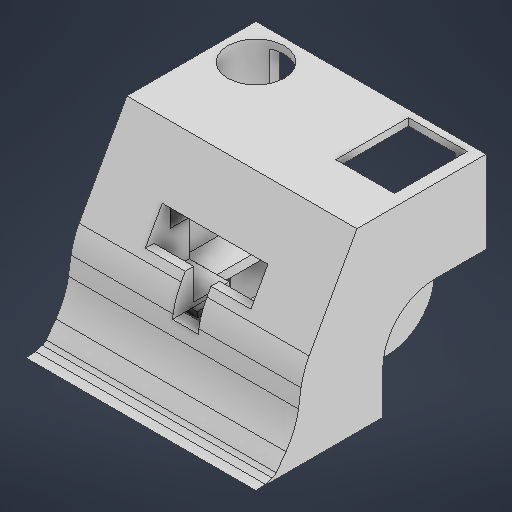
# Autodesk Inventor part: najlepszetrzecieniepierwszekolokwium
Saved by Autodesk Inventor 2026 (Build 300175000, 175)
## iProperties
Created: 2025-12-31
Part Number: najlepszetrzecieniepierwszekolokwium
Material: Ogólny
Document SubType Name: Modeling
Designer: macie
Density: 1 g/cm^3
Appearance: Domyślna
Author: macie
Autodesk Inventor part; units mm, degrees
ref_plane "YZ Plane" through (0, 0, 0) normal (1, 0, 0) x (0, 1, 0)
ref_plane "XZ Plane" through (0, 0, 0) normal (0, 1, 0) x (-1, 0, 0)
ref_plane "XY Plane" through (0, 0, 0) normal (0, 0, 1) x (1, 0, 0)
sketch "Szkic1" plane through (0, 0, 0) normal (0, 1, 0) x (-1, 0, 0)
  line L0 (49, 49) -> (-49, 49)
  line L1 (-49, 49) -> (-49, -49)
  line L2 (-49, -49) -> (49, -49)
  line L3 (49, -49) -> (49, 49)
  line L4 (49, 49) -> (-49, -49) construction
  line L5 (-49, 49) -> (49, -49) construction
  point P0 (0, 0)
  dimension "d0" = 98
  dimension "d1" = 98
  constraints: 12 end point, 2 midpoint, 2 parallel, 1 horizontal, 1 perpendicular
  measures "d0" distance between parallel lines of L1 L3
  measures "d1" distance between parallel lines of L2 L0
extrude "Wyciągnięcie proste1" add sketch "Szkic1" along normal blind 98
sketch "Szkic2" plane through (49, 0, 49) normal (1, 0, 0) x (0, 0, -1)
  line L0 (0, 0) -> (98, 0) projected
  line L1 (98, 0) -> (76, 0)
  line L2 (76, 0) -> (76, 18)
  circle A0 centre (76, 18) radius 22
  line L3 (98, 0) -> (98, 98) projected
  line L4 (98, 18) -> (98, 0)
  line L5 (98, 0) -> (88.6491, 0)
  line L6 (76, 40) -> (98, 40)
  line L7 (98, 18) -> (98, 40)
  line L8 (54, 18) -> (54, 0)
  line L9 (63.3509, 0) -> (54, 0)
  point P0 (49, 0)
  dimension "d4" = 22
  dimension "d5" = 18
  dimension "d6" = 44
  constraints: 16 end point, 6 point on line, 5 point on circle, 2 collinear, 2 perpendicular, 2 tangent, 2 vertical, 1 centre point, 1 coincident
  measures "d4" distance of L0.end L1.end
  measures "d5" distance of L1.end L2.end
  measures "d6" diameter of A0
extrude "Wyciągnięcie proste2" cut sketch "Szkic2" against normal blind 98 contours L8 A0 L0 | A0 L0 | A0 L3 L0 | L6 L3 A0 picked at (77.6318, 26.4828)
sketch "Szkic3" plane through (0, 0, 0) normal (0, -1, 0) x (1, 0, 0)
  line L0 (49, -49) -> (-49, -49) projected
  line L1 (49, -49) -> (27, -49)
  line L2 (-49, -49) -> (-27, -49)
  line L3 (-49, -5) -> (49, -5) projected
  line L4 (-27, -49) -> (27, -49)
  line L5 (27, -49) -> (27, -5)
  line L6 (27, -5) -> (-27, -5)
  line L7 (-27, -5) -> (-27, -49)
  point P0 (0, 0)
  dimension "d10" = 22
  dimension "d11" = 22
  dimension "d12" = 54
  constraints: 12 end point, 3 point on line, 2 parallel, 1 horizontal, 1 perpendicular
  measures "d10" distance of L1.end L0.start
  measures "d11" distance of L2.end L0.end
  measures "d12" distance between parallel lines of L7 L5
extrude "Wyciągnięcie proste3" add sketch "Szkic3" against normal blind 40
sketch "Szkic4" plane through (27, 0, -5) normal (1, 0, 0) x (0, 0, -1)
  line L0 (44, 0) -> (44, 40) projected
  line L1 (44, 18) -> (44, 0)
  line L2 (44, 18) -> (22, 18)
  line L3 (22, 12) -> (22, 24)
  line L4 (15, 24) -> (29, 24)
  line L5 (15, 24) -> (15, 12)
  line L6 (15, 12) -> (29, 12)
  line L7 (29, 12) -> (29, 24)
  point P0 (-5, 0)
  dimension "d15" = 18
  dimension "d16" = 22
  dimension "d17" = 12
  dimension "d18" = 14
  dimension "d19" = 12
  constraints: 14 end point, 3 vertical, 2 horizontal, 2 midpoint, 2 perpendicular, 1 point on line
  measures "d15" distance of L0.start L1.start
  measures "d16" distance of L1.start L2.end
  measures "d17" distance of L3.start L3.end
  measures "d18" distance of L4.end L4.start
  measures "d19" distance between parallel lines of L4 L6
extrude "Wyciągnięcie proste4" cut sketch "Szkic4" against normal through all
sketch "Szkic5" plane through (49, 98, -49) normal (0, 0, -1) x (-1, 0, 0)
  line L0 (98, 0) -> (0, 0) projected
  line L1 (98, -98) -> (98, 0) projected
  line L2 (0, 0) -> (98, 0)
  line L3 (98, 0) -> (98, -30)
  line L4 (98, -30) -> (0, -30)
  line L5 (0, -30) -> (0, 0)
  line L6 (0, -58) -> (22, -58) projected
  line L7 (10, -58) -> (88, -58)
  line L8 (88, -58) -> (88, -38)
  line L9 (88, -38) -> (10, -38)
  line L10 (10, -38) -> (10, -58)
  line L11 (0, -58) -> (0, 0) projected
  line L12 (22, -86) -> (76, -86) projected
  line L13 (38, -86) -> (60, -86)
  line L14 (60, -86) -> (60, -58)
  line L15 (60, -58) -> (38, -58)
  line L16 (38, -58) -> (38, -86)
  line L17 (22, -98) -> (22, -58) projected
  line L18 (76, -98) -> (76, -58) projected
  line L19 (22, -70) -> (38, -70)
  line L20 (60, -70) -> (76, -70)
  line L21 (76, -70) -> (76, -58)
  line L22 (22, -70) -> (22, -58)
  line L23 (22, -74) -> (76, -74) projected
  line L24 (22, -90) -> (22, -96)
  line L25 (76, -96) -> (22, -96)
  line L26 (76, -96) -> (76, -86)
  line L27 (76, -98) -> (22, -98) projected
  line L28 (22, -96) -> (22, -90)
  line L29 (22, -90) -> (76, -90)
  line L30 (76, -96) -> (76, -90)
  line L31 (38, -86) -> (38, -90)
  line L32 (60, -86) -> (60, -90)
  line L33 (24, -58) -> (24, -70)
  line L34 (74, -58) -> (74, -70)
  line L35 (10, -56) -> (24, -56)
  line L36 (24, -56) -> (24, -58)
  line L37 (74, -58) -> (74, -56)
  line L38 (74, -56) -> (88, -56)
  point P0 (49, -98)
  dimension "d22" = 30
  dimension "d23" = 20
  dimension "d25" = 10
  dimension "d26" = 10
  dimension "d27" = 16
  dimension "d28" = 16
  dimension "d29" = 4
  dimension "d30" = 2
  dimension "d31" = 4
  dimension "d32" = 2
  dimension "d33" = 2
  dimension "d34" = 2
  dimension "d35" = 2
  constraints: 60 end point, 22 point on line, 13 perpendicular, 6 parallel, 5 collinear, 2 horizontal, 1 vertical
  measures "d22" distance between parallel lines of L4 L0
  measures "d23" distance between parallel lines of L7 L9
  measures "d25" distance between parallel lines of L11 L10
  measures "d26" distance between parallel lines of L1 L8
  measures "d27" distance between parallel lines of L17 L16
  measures "d28" distance between parallel lines of L18 L14
  measures "d29" distance between parallel lines of L23 L19
  measures "d30" distance between parallel lines of L27 L25
  measures "d31" distance between parallel lines of L29 L12
  measures "d32" distance between parallel lines of L17 L33
  measures "d33" distance between parallel lines of L34 L18
  measures "d34" distance between parallel lines of L7 L35
  measures "d35" distance between parallel lines of L7 L38
extrude "Wyciągnięcie proste5" cut sketch "Szkic5" against normal blind 55 contours L10 L9 L8 L38 L37 L7 L36 L35 | L7 L16 L19 L33 | L7 L14 L23 L16 | L7 L34 L20 L14 | L23 L14 L12 L16
sketch "Szkic6" plane through (0, 0, 0) normal (0, -1, 0) x (1, 0, 0)
  line L0 (38.5, -16) -> (-38.5, -16)
  line L1 (-38.5, -16) -> (-38.5, 25)
  line L2 (-38.5, 25) -> (38.5, 25)
  line L3 (38.5, 25) -> (38.5, -16)
  line L4 (-49, -5) -> (-49, 49) projected
  line L5 (49, 49) -> (49, -5) projected
  line L6 (27, -5) -> (49, -5) projected
  line L7 (27, -20) -> (11, -20) projected
  point P0 (0, 0)
  dimension "d38" = 41
  dimension "d40" = 10.5
  dimension "d41" = 10.5
  dimension "d45" = 4
  constraints: 8 end point, 2 parallel, 1 horizontal, 1 perpendicular
  measures "d38" distance between parallel lines of L2 L0
  measures "d40" distance between parallel lines of L4 L1
  measures "d41" distance between parallel lines of L3 L5
  measures "d45" distance between parallel lines of L0 L7
extrude "Wyciągnięcie proste6" cut sketch "Szkic6" against normal blind 24
sketch "Szkic7" plane through (0, 0, 0) normal (0, -1, 0) x (1, 0, 0)
  line L0 (-38.5, 25) -> (38.5, 25) projected
  line L1 (38.5, 25) -> (29.5, 25)
  line L2 (29.5, 25) -> (29.5, 39)
  line L3 (29.5, 39) -> (38.5, 39)
  line L4 (38.5, 39) -> (38.5, 25)
  line L5 (-38.5, 25) -> (-29.5, 25)
  line L6 (-29.5, 25) -> (-29.5, 39)
  line L7 (-29.5, 39) -> (-38.5, 39)
  line L8 (-38.5, 39) -> (-38.5, 25)
  point P0 (0, 0)
  point P1 (-38.5, 32)
  point P2 (-29.5, 32)
  dimension "d46" = 14
  dimension "d47" = 14
  dimension "d48" = 9
  dimension "d49" = 9
  constraints: 16 end point, 4 parallel, 2 midpoint, 2 perpendicular, 2 point on line
  measures "d46" distance between parallel lines of L3 L0
  measures "d47" distance between parallel lines of L7 L0
  measures "d48" distance between parallel lines of L2 L4
  measures "d49" distance of point (-38.5, 32) point (-29.5, 32)
extrude "Wyciągnięcie proste7" cut sketch "Szkic7" against normal blind 3.5
sketch "Szkic8" plane through (0, 3.5, 0) normal (0, -1, 0) x (1, 0, 0)
  line L0 (-38.5, 25) -> (38.5, 25) projected
  line L1 (38.5, 25) -> (35.5, 25)
  line L2 (35.5, 25) -> (35.5, 27)
  line L3 (35.5, 27) -> (38.5, 27)
  line L4 (38.5, 27) -> (38.5, 25)
  line L5 (-38.5, -5) -> (-38.5, 39) projected
  line L6 (-38.5, 25) -> (-38.5, 27)
  line L7 (-38.5, 27) -> (-35.5, 27)
  line L8 (-35.5, 27) -> (-35.5, 25)
  line L9 (-35.5, 25) -> (-38.5, 25)
  point P0 (0, 0)
  point P1 (38.5, 26)
  point P2 (35.5, 26)
  point P3 (37, 25)
  point P4 (37, 27)
  point P5 (-38.5, 26)
  point P6 (-37, 25)
  point P7 (-37, 27)
  dimension "d52" = 3
  dimension "d53" = 2
  dimension "d54" = 3
  dimension "d55" = 2
  constraints: 16 end point, 7 midpoint, 4 parallel, 2 perpendicular, 2 point on line
  measures "d52" distance of point (38.5, 26) point (35.5, 26)
  measures "d53" distance of point (37, 25) point (37, 27)
  measures "d54" distance from line of point (-38.5, 26) L8
  measures "d55" distance of point (-37, 25) point (-37, 27)
extrude "Wyciągnięcie proste8" cut sketch "Szkic8" against normal blind 23
sketch "Szkic9" plane through (0, 24, 0) normal (0, -1, 0) x (1, 0, 0)
  line L0 (38.5, 27) -> (38.5, 25) projected
  line L1 (-38.5, -5) -> (-38.5, 39) projected
  line L2 (38.5, 25) -> (-38.5, 25)
  line L3 (-38.5, 25) -> (-38.5, 22)
  line L4 (-38.5, 22) -> (38.5, 22)
  line L5 (38.5, 22) -> (38.5, 25)
  point P0 (0, 0)
  dimension "d58" = 3
  constraints: 8 end point, 2 parallel, 1 horizontal, 1 perpendicular, 1 point on line
  measures "d58" distance between parallel lines of L2 L4
extrude "Wyciągnięcie proste9" cut sketch "Szkic9" against normal blind 2.5
sketch "Szkic10" plane through (0, 24, 0) normal (0, -1, 0) x (1, 0, 0)
  line L0 (11, 6) -> (-11, 6) projected
  line L1 (38.5, 22) -> (-38.5, 22) projected
  line L2 (3, 6) -> (3, 22)
  line L3 (3, 22) -> (-3, 22)
  line L4 (-3, 22) -> (-3, 6)
  line L5 (-3, 6) -> (3, 6)
  line L6 (11, -16) -> (11, 6) projected
  point P0 (0, 0)
  point P1 (-3, 6)
  dimension "d61" = 6
  dimension "d62" = 8
  constraints: 8 end point, 2 parallel, 2 point on line, 1 perpendicular, 1 vertical
  measures "d61" distance between parallel lines of L4 L2
  measures "d62" distance between parallel lines of L6 L2
extrude "Wyciągnięcie proste10" cut sketch "Szkic10" against normal blind 2.5
sketch "Szkic11" plane through (49, 0, 49) normal (1, 0, 0) x (0, 0, -1)
  line L0 (54, 0) -> (0, 0) projected
  line L1 (0, 0) -> (4, 0.35)
  line L2 (4, 0.35) -> (8, 1.4218)
  line L3 (8, 1.4218) -> (17, 13.8812)
  line L4 (17, 13.8812) -> (20, 33.6621)
  line L5 (20, 33.6621) -> (43, 75.12)
  line L6 (43, 75.12) -> (98, 75.12)
  line L7 (98, 40) -> (98, 98) projected
  line L8 (0, 0) -> (0, 98) projected
  line L9 (0, 0) -> (0, 98)
  line L10 (98, 98) -> (0, 98) projected
  line L11 (0, 98) -> (98, 98)
  line L12 (98, 98) -> (98, 75.12)
  point P0 (49, 0)
  dimension "d65" = 5
  dimension "d66" = 4
  dimension "d67" = 15
  dimension "d68" = 4
  dimension "d69" = 54.158
  dimension "d70" = 81.376
  dimension "d71" = 60.979
  dimension "d72" = 20
  dimension "d73" = 3
  dimension "d74" = 55
  constraints: 18 end point, 2 perpendicular, 1 collinear, 1 horizontal, 1 point on line
  measures "d65" angle of L0 L1
  measures "d66" horizontal distance of L0.end L1.end
  measures "d67" angle of L0 L2
  measures "d68" horizontal distance of L2.end L1.end
  measures "d69" angle of L0 L3
  measures "d70" angle of L0 L4
  measures "d71" angle of L0 L5
  measures "d72" horizontal distance of L0.end L4.end
  measures "d73" horizontal distance of L4.end L3.end
  measures "d74" distance of L6.end L5.end
extrude "Wyciągnięcie proste11" cut sketch "Szkic11" against normal through all
sketch "Szkic12" plane through (0, 26.5, 0) normal (0, -1, 0) x (1, 0, 0)
  line L0 (3, 22) -> (3, 6) projected
  line L1 (-3, 6) -> (-3, 22) projected
  line L2 (3, 22) -> (-3, 22)
  line L3 (-3, 22) -> (-3, 25)
  line L4 (-3, 25) -> (3, 25)
  line L5 (3, 25) -> (3, 22)
  point P0 (0, 0)
  constraints: 8 end point, 2 parallel, 1 horizontal, 1 perpendicular
extrude "Wyciągnięcie proste12" cut sketch "Szkic12" against normal blind 15
sketch "Szkic13" plane through (49, 98, 6) normal (0, 0, -1) x (-1, 0, 0)
  line L0 (52, -71.5) -> (87.5, -71.5) projected
  line L1 (54.5, -71.5) -> (54.5, -57.4075)
  line L2 (46, -71.5) -> (13.5, -71.5) projected
  line L3 (43.5, -71.5) -> (43.5, -56.5)
  line L4 (38, -86) -> (38, -70) projected
  line L5 (60, -70) -> (60, -86) projected
  line L6 (43.5, -56.5) -> (26.5, -56.5)
  line L7 (26.5, -56.5) -> (26.5, -43.5)
  line L8 (26.5, -43.5) -> (71.5, -43.5)
  line L9 (71.5, -43.5) -> (71.5, -56.5)
  line L10 (71.5, -56.5) -> (54.5, -56.5)
  line L11 (54.5, -56.5) -> (54.5, -57.4075)
  line L12 (43.5, -71.5) -> (54.5, -71.5)
  point P0 (49, -98)
  dimension "d80" = 5.5
  dimension "d81" = 5.5
  dimension "d82" = 17
  dimension "d83" = 17
  dimension "d84" = 13
  dimension "d85" = 15
  constraints: 18 end point, 4 perpendicular, 4 point on line, 2 horizontal, 2 vertical
  measures "d80" distance between parallel lines of L3 L4
  measures "d81" distance between parallel lines of L5 L1
  measures "d82" distance between parallel lines of L7 L3
  measures "d83" distance between parallel lines of L9 L1
  measures "d84" distance between parallel lines of L8 L6
  measures "d85" distance between parallel lines of L2 L6
extrude "Wyciągnięcie proste13" cut sketch "Szkic13" against normal through all
sketch "Szkic14" plane through (49, 75.12, 6) normal (0, 1, 0) x (1, 0, 0)
  line L0 (-10, 55) -> (-10, 0) projected
  line L1 (-10, 52) -> (-30, 52)
  line L2 (-30, 52) -> (-30, 21)
  line L3 (-30, 21) -> (-10, 21)
  line L4 (-10, 21) -> (-10, 52)
  line L5 (-98, 55) -> (0, 55) projected
  circle A0 centre (-83, 40) radius 12
  line L6 (-98, 0) -> (-98, 55) projected
  line L7 (-10, 52) -> (-5, 52)
  line L8 (-5, 52) -> (-5, 21)
  line L9 (-5, 21) -> (-10, 21)
  line L10 (-10, 21) -> (-10, 52)
  point P0 (-49, 6)
  point P1 (-7.5, 21)
  point P2 (-7.5, 52)
  point P3 (-10, 21)
  dimension "d88" = 20
  dimension "d89" = 31
  dimension "d90" = 3
  dimension "d91" = 24
  dimension "d92" = 15
  dimension "d93" = 15
  dimension "d94" = 5
  dimension "d95" = 31
  constraints: 16 end point, 4 parallel, 2 horizontal, 2 midpoint, 2 perpendicular, 1 centre point, 1 point on line
  measures "d88" distance between parallel lines of L2 L0
  measures "d89" distance between parallel lines of L1 L3
  measures "d90" distance between parallel lines of L5 L1
  measures "d91" diameter of A0
  measures "d92" distance from line of L6 A0.centre
  measures "d93" distance from line of L5 A0.centre
  measures "d94" distance between parallel lines of L8 L0
  measures "d95" distance of point (-7.5, 21) point (-7.5, 52)
extrude "Wyciągnięcie proste14" cut sketch "Szkic14" against normal blind 27
fillet "Zaokrąglenie1" radius 30 2 edges at (27.25, 33.6621, 29) (-27.25, 33.6621, 29)
fillet "Zaokrąglenie2" radius 30 1 edges at (0, 13.8812, 32)
fillet "Zaokrąglenie3" radius 3 1 edges at (0, 1.4218, 41)
fillet "Zaokrąglenie4" radius 20 1 edges at (0, 0, -49)
sketch "Szkic15" plane through (-27, 40, -49) normal (0, 0, -1) x (-1, 0, 0)
  line L0 (-66, 8.12) -> (-66, 20) projected
  line L1 (12, 20) -> (-5, 20) projected
  line L2 (-66, 20) -> (12, 20)
  line L3 (12, 20) -> (12, 32)
  line L4 (12, 32) -> (-66, 32)
  line L5 (-66, 32) -> (-66, 20)
  point P0 (-27, -40)
  dimension "d102" = 12
  constraints: 8 end point, 2 parallel, 1 collinear, 1 perpendicular
  measures "d102" distance between parallel lines of L2 L4
extrude "Wyciągnięcie proste15" cut sketch "Szkic15" against normal blind 55
sketch "Szkic16" plane through (49, 98, 6) normal (0, 0, -1) x (-1, 0, 0)
  line L0 (26.5, -56.5) -> (26.5, -43.5) projected
  line L1 (71.5, -43.5) -> (26.5, -43.5) projected
  line L2 (26.5, -43.5) -> (71.5, -43.5)
  line L3 (71.5, -43.5) -> (71.5, -35.5)
  line L4 (71.5, -35.5) -> (26.5, -35.5)
  line L5 (26.5, -35.5) -> (26.5, -43.5)
  line L6 (98, -69.6738) -> (54.5, -69.6738) projected
  line L7 (71.5, -56.5) -> (54.5, -56.5) projected
  line L8 (54.5, -69.6738) -> (54.5, -56.5)
  line L9 (54.5, -56.5) -> (71.5, -56.5)
  line L10 (71.5, -56.5) -> (71.5, -69.6738)
  line L11 (71.5, -69.6738) -> (54.5, -69.6738)
  line L12 (26.5, -56.5) -> (43.5, -56.5) projected
  line L13 (43.5, -56.5) -> (43.5, -69.6738)
  line L14 (43.5, -69.6738) -> (26.5, -69.6738)
  line L15 (26.5, -69.6738) -> (26.5, -56.5)
  line L16 (26.5, -56.5) -> (43.5, -56.5)
  line L17 (10, -56) -> (10, -26) projected
  line L18 (10, -35.5) -> (26.5, -35.5)
  line L19 (26.5, -35.5) -> (26.5, -55)
  line L20 (26.5, -55) -> (10, -55)
  line L21 (10, -55) -> (10, -35.5)
  line L22 (88, -26) -> (88, -56) projected
  line L23 (71.5, -35.5) -> (88, -35.5)
  line L24 (88, -35.5) -> (88, -55)
  line L25 (88, -55) -> (71.5, -55)
  line L26 (71.5, -55) -> (71.5, -35.5)
  line L27 (24, -56) -> (10, -56) projected
  line L28 (88, -56) -> (74, -56) projected
  line L29 (43.5, -71.5) -> (43.5, -56.5) projected
  point P0 (49, -98)
  point P1 (43.5, -64)
  point P2 (54.5, -63.0869)
  dimension "d105" = 8
  dimension "d106" = 1
  dimension "d107" = 1
  dimension "d108" = 17
  dimension "d109" = 17
  constraints: 40 end point, 11 parallel, 7 perpendicular, 4 point on line, 2 midpoint, 1 collinear
  measures "d105" distance between parallel lines of L1 L4
  measures "d106" distance between parallel lines of L27 L20
  measures "d107" distance between parallel lines of L28 L25
  measures "d108" distance from line of point (43.5, -64) L15
  measures "d109" distance from line of L10 point (54.5, -63.087)
extrude "Wyciągnięcie proste16" cut sketch "Szkic16" against normal blind 15 contours L6 L8 L7 L10 | L12 L13 L14 L15
sketch "Szkic17" plane through (49, 98, 6) normal (0, 0, -1) x (-1, 0, 0)
  line L0 (26.5, -43.5) -> (26.5, -56.5) projected
  line L1 (26.5, -43.5) -> (71.5, -43.5) projected
  line L2 (26.5, -54.5) -> (26.5, -43.5)
  line L3 (26.5, -43.5) -> (11.5, -43.5)
  line L4 (11.5, -43.5) -> (11.5, -54.5)
  line L5 (11.5, -54.5) -> (26.5, -54.5)
  line L6 (71.5, -43.5) -> (71.5, -54.5)
  line L7 (71.5, -54.5) -> (86.5, -54.5)
  line L8 (86.5, -54.5) -> (86.5, -43.5)
  line L9 (86.5, -43.5) -> (71.5, -43.5)
  point P0 (49, -98)
  point P1 (79, -54.5)
  point P2 (19, -43.5)
  point P3 (19, -54.5)
  dimension "d112" = 15
  dimension "d113" = 15
  dimension "d114" = 11
  dimension "d115" = 11
  constraints: 16 end point, 4 parallel, 4 perpendicular, 3 midpoint, 1 point on line
  measures "d112" distance between parallel lines of L0 L4
  measures "d113" distance between parallel lines of L8 L6
  measures "d114" distance from line of L9 point (79, -54.5)
  measures "d115" distance of point (19, -43.5) point (19, -54.5)
extrude "Wyciągnięcie proste17" cut sketch "Szkic17" against normal blind 8
sketch "Szkic18" plane through (49, 98, 6) normal (0, 0, -1) x (-1, 0, 0)
  line L0 (11.5, -54.5) -> (11.5, -43.5) projected
  line L1 (86.5, -43.5) -> (86.5, -54.5) projected
  line L2 (11.5, -43.5) -> (86.5, -43.5)
  line L3 (86.5, -43.5) -> (86.5, -31.5)
  line L4 (86.5, -31.5) -> (11.5, -31.5)
  line L5 (11.5, -31.5) -> (11.5, -43.5)
  point P0 (49, -98)
  dimension "d118" = 12
  constraints: 8 end point, 2 parallel, 1 horizontal, 1 perpendicular
  measures "d118" distance between parallel lines of L4 L2
extrude "Wyciągnięcie proste18" cut sketch "Szkic18" against normal blind 3
fillet "Zaokrąglenie5" radius 10 1 edges at (0, 54.5, 9)
fillet "Zaokrąglenie6" radius 2 1 edges at (37.5, 55, 6)
fillet "Zaokrąglenie7" radius 2 1 edges at (-37.5, 55, 6)
equation "\"d41\" = d40"
equation "\"d47\" = d46"
equation "\"d49\" = d48"
equation "\"d54\" = d52"
equation "\"d55\" = d53"
equation "\"d81\" = d80"
